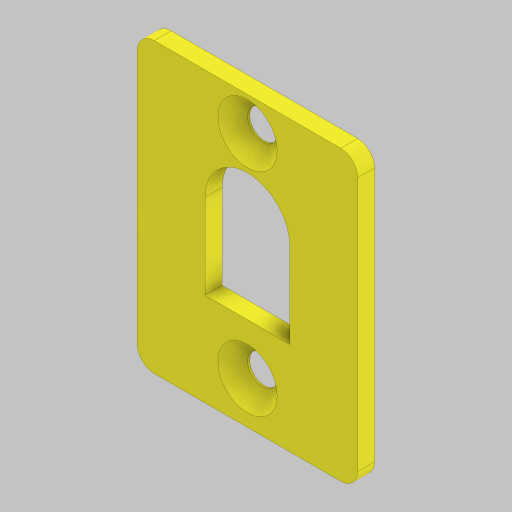
# Autodesk Inventor part: Rückwand Deckplatte
Saved by Autodesk Inventor 2023 (Build 270158030, 158C)
## iProperties
Created: 2022-09-18
Part Number: Rückwand Deckplatte
Material: PVC, hart
Document SubType Name: Modeling
Designer: musati
Density: 1.29 g/cm^3
Appearance: Kanariengelb
Author: musati
Autodesk Inventor part; units mm, degrees
ref_plane "YZ Plane" through (0, 0, 0) normal (1, 0, 0) x (0, 1, 0)
ref_plane "XZ Plane" through (0, 0, 0) normal (0, 1, 0) x (-1, 0, 0)
ref_plane "XY Plane" through (0, 0, 0) normal (0, 0, 1) x (1, 0, 0)
sketch "Skizze1" plane through (0, 0, 0) normal (0, 0, 1) x (1, 0, 0)
  line L0 (-18.7799, 0) -> (18.7799, 0) projected
  line L1 (0, -24.3799) -> (0, 24.3799) projected
  line L2 (-11, -17) -> (11, -17)
  line L3 (13, -15) -> (13, 15)
  line L4 (11, 17) -> (-11, 17)
  line L5 (-13, 15) -> (-13, -15)
  line L6 (-13, -17) -> (13, 17) construction
  line L7 (13, -17) -> (-13, 17) construction
  arc A0 (-11, 17) -> (-13, 15) centre (-11, 15) ccw
  arc A1 (13, 15) -> (11, 17) centre (11, 15) ccw
  arc A2 (11, -17) -> (13, -15) centre (11, -15) ccw
  arc A3 (-13, -15) -> (-11, -17) centre (-11, -15) ccw
  point P0 (0, 0)
  dimension "d0" = 26
  dimension "d1" = 34
  dimension "d2" = 2
  constraints: 12 end point, 8 point on circle, 8 point on line, 8 tangent, 4 centre point, 3 equal radius, 2 midpoint, 2 parallel, 1 horizontal, 1 perpendicular
  measures "d0" distance of L7.end L6.end
  measures "d1" distance of L6.end L7.start
  measures "d2" radius of A0
extrude "Extrusion1" add sketch "Skizze1" against normal blind 2
sketch "Skizze2" plane through (0, 0, 0) normal (0, 0, 1) x (1, 0, 0)
  line L0 (13, -15) -> (13, 15) projected
  arc A0 (13, 15) -> (11, 17) centre (11, 15) ccw projected
  line L1 (11, 17) -> (-11, 17) projected
  arc A1 (-11, 17) -> (-13, 15) centre (-11, 15) ccw projected
  line L2 (-13, 15) -> (-13, -15) projected
  arc A2 (-13, -15) -> (-11, -17) centre (-11, -15) ccw projected
  line L3 (-11, -17) -> (11, -17) projected
  arc A3 (11, -17) -> (13, -15) centre (11, -15) ccw projected
  line L4 (-18.7799, 0) -> (18.7799, 0) projected
  line L5 (0, -24.3799) -> (0, 24.3799) projected
  line L6 (-5, 4) -> (5, 4)
  line L7 (5, 4) -> (5, -6)
  line L8 (5, -6) -> (-5, -6)
  line L9 (-5, -6) -> (-5, 4)
  arc A4 (5, 4) -> (-5, 4) centre (0, 4) ccw
  point P0 (0, 0)
  dimension "d5" = 10
  dimension "d6" = 10
  dimension "d7" = 11
  dimension "d8" = 5
  constraints: 8 end point, 2 parallel, 2 point on circle, 1 centre point, 1 horizontal, 1 perpendicular, 1 other
  measures "d5" distance of L7.end L8.end
  measures "d6" distance of L6.end L7.end
  measures "d7" distance between parallel lines of L8 L3
  measures "d8" radius of A4
extrude "Extrusion2" cut sketch "Skizze2" against normal blind 2 contours L7 L8 L5 L4 | L4 L5 L6 L7 | L5 L8 L9 L4 | L4 L9 L6 L5 | L6 L5 A4 | L6 A4 L5
sketch "Skizze3" plane through (0, 0, 0) normal (0, 0, 1) x (1, 0, 0)
  line L0 (5, 4) -> (5, -6) projected
  line L1 (5, -6) -> (-5, -6) projected
  line L2 (-5, -6) -> (-5, 4) projected
  arc A0 (5, 4) -> (-5, 4) centre (0, 4) ccw projected
  line L3 (13, -15) -> (13, 15) projected
  arc A1 (13, 15) -> (11, 17) centre (11, 15) ccw projected
  line L4 (11, 17) -> (-11, 17) projected
  arc A2 (-11, 17) -> (-13, 15) centre (-11, 15) ccw projected
  line L5 (-13, 15) -> (-13, -15) projected
  arc A3 (-13, -15) -> (-11, -17) centre (-11, -15) ccw projected
  line L6 (-11, -17) -> (11, -17) projected
  arc A4 (11, -17) -> (13, -15) centre (11, -15) ccw projected
  line L7 (-18.7799, 0) -> (18.7799, 0) projected
  line L8 (0, -24.3799) -> (0, 24.3799) projected
  point P0 (0, 0)
  point P1 (0, -12)
  point P2 (0, 13)
  dimension "d11" = 25
  dimension "d12" = 5
  constraints: 2 point on line
  measures "d11" distance of point (0, 13) point (0, -12)
  measures "d12" distance from line of point (0, -12) L6
hole "Bohrung1" at (0, -12, 0) at (0, 13, 0) direction (0, 0, -1) diameter 3.5 end through all countersink diameter 7 countersink angle 90
